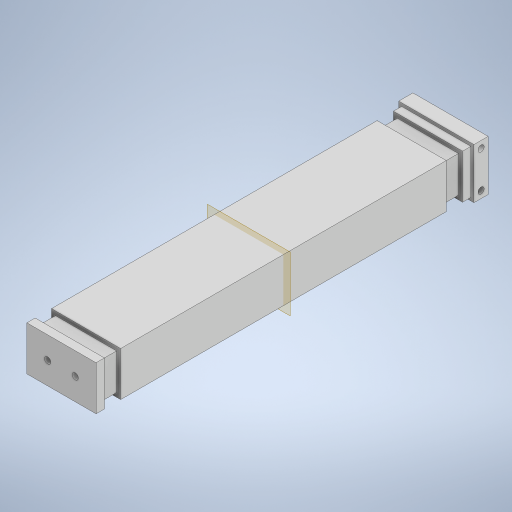
# Autodesk Inventor part: Mold
Saved by Autodesk Inventor 2024 (Build 280153000, 153)
## iProperties
Created: 2024-09-09
Part Number: Mold
Material: Generic
Document SubType Name: Modeling
Designer: Bruger
Density: 1 g/cm^3
Appearance: Default
Author: Bruger
Autodesk Inventor part; units mm, degrees
ref_plane "YZ Plane" through (0, 0, 0) normal (1, 0, 0) x (0, 1, 0)
ref_plane "XZ Plane" through (0, 0, 0) normal (0, 1, 0) x (-1, 0, 0)
ref_plane "XY Plane" through (0, 0, 0) normal (0, 0, 1) x (1, 0, 0)
sketch "Sketch8" plane through (0, 0, 0) normal (0, 0, 1) x (1, 0, 0)
  line L0 (-18.5, -12.375) -> (18.5, -12.375)
  line L1 (18.5, -12.375) -> (18.5, 12.375)
  line L2 (18.5, 12.375) -> (-18.5, 12.375)
  line L3 (-18.5, 12.375) -> (-18.5, -12.375)
  line L4 (-18.5, -12.375) -> (18.5, 12.375) construction
  line L5 (18.5, -12.375) -> (-18.5, 12.375) construction
  point P0 (0, 0)
  dimension "d43" = 37
  dimension "d44" = 24.75
  constraints: 12 end point, 2 midpoint, 2 parallel, 1 horizontal, 1 perpendicular
  measures "d43" distance of L2.end L1.end
  measures "d44" distance of L1.end L0.end
extrude "Extrusion6" add sketch "Sketch8" along normal blind 7
sketch "Sketch9" plane through (0, 0, 7) normal (0, 0, 1) x (1, 0, 0)
  line L0 (-17, -10.875) -> (17, -10.875)
  line L1 (17, -10.875) -> (17, 10.875)
  line L2 (17, 10.875) -> (-17, 10.875)
  line L3 (-17, 10.875) -> (-17, -10.875)
  line L4 (-17, -10.875) -> (17, 10.875) construction
  line L5 (17, -10.875) -> (-17, 10.875) construction
  line L6 (18.5, 12.375) -> (-18.5, 12.375) projected
  line L7 (18.5, -12.375) -> (18.5, 12.375) projected
  point P0 (0, 0)
  dimension "d49" = 1.5
  dimension "d50" = 1.5
  constraints: 12 end point, 2 midpoint, 2 parallel, 1 horizontal, 1 perpendicular
  measures "d49" distance between parallel lines of L6 L2
  measures "d50" distance between parallel lines of L7 L1
extrude "Extrusion7" add sketch "Sketch9" along normal blind 184.3
sketch "Sketch10" plane through (18.5, -12.375, 0) normal (1, 0, 0) x (0, 0, -1)
  circle A0 centre (-3.5, 21.325) radius 1.5
  line L0 (0, 0) -> (0, 24.75) projected
  line L1 (0, 24.75) -> (-7, 24.75) projected
  point P0 (0, 12.375)
  dimension "d53" = 3
  dimension "d56" = 3.425
  dimension "d57" = 3.5
  constraints: 1 centre point
  measures "d53" diameter of A0
  measures "d56" distance from line of L1 A0.centre
  measures "d57" distance from line of L0 A0.centre
hole "Hole1" at (18.5, 8.95, 3.5) direction (-1, 0, 0) diameter 3 depth 5 tip angle 118
mirror "Mirror1" about plane through (0, 0, 0) normal (0, 1, 0) of "Hole1"
mirror "Mirror2" about plane through (0, 0, 0) normal (1, 0, 0) of "Hole1", "Mirror1"
sketch "Sketch11" plane through (-18.5, -12.375, 0) normal (0, -1, 0) x (1, 0, 0)
  line L0 (18.5, 0) -> (18.5, 7)
  line L1 (37, 7) -> (0, 7) projected
  line L2 (18.5, 3.5) -> (0, 3.5)
  line L3 (0, 0) -> (0, 7) projected
  circle A0 centre (9.25, 3.5) radius 1.5
  dimension "d66" = 3
  constraints: 4 end point, 4 midpoint, 1 centre point
  measures "d66" diameter of A0
hole "Hole2" at (-9.25, -12.375, 3.5) direction (0, 1, 0) diameter 3 depth 5 tip angle 118
mirror "Mirror3" about plane through (0, 0, 0) normal (1, 0, 0) of "Hole2"
sketch "Sketch12" plane through (0, 0, 191.3) normal (0, 0, 1) x (1, 0, 0)
  circle A0 centre (6.8, 0) radius 1.5
  line L0 (17, -10.875) -> (17, 10.875) projected
  line L1 (17, 10.875) -> (-17, 10.875) projected
  point P0 (0, 0)
  dimension "d74" = 3
  dimension "d75" = 10.2
  dimension "d76" = 10.875
  constraints: 1 centre point
  measures "d74" diameter of A0
  measures "d75" distance from line of L0 A0.centre
  measures "d76" distance from line of L1 A0.centre
hole "Hole3" at (6.8, 0, 191.3) direction (0, 0, -1) diameter 3 depth 5 tip angle 118
mirror "Mirror4" about plane through (0, 0, 0) normal (1, 0, 0) of "Hole3"
sketch "Sketch13" plane through (-17, -10.875, 7) normal (-1, 0, 0) x (0, 0, 1)
  line L0 (0, 21.75) -> (4.1, 21.75)
  line L1 (0, 21.75) -> (184.3, 21.75) projected
  line L2 (4.1, 21.75) -> (4.1, 0)
  line L3 (0, 0) -> (184.3, 0) projected
  line L4 (4.1, 21.75) -> (12.1, 21.75)
  line L5 (0, 21.75) -> (184.3, 21.75) projected
  line L6 (12.1, 21.75) -> (12.1, 0)
  line L7 (12.1, 0) -> (4.1, 0)
  point P0 (-7, 10.875)
  dimension "d84" = 4.1
  dimension "d85" = 90
  dimension "d86" = 8
  dimension "d87" = 90
  constraints: 10 end point, 4 point on line
  measures "d84" distance of L0.start L0.end
  measures "d85" angle of L0 L2
  measures "d86" distance of L0.end L4.end
  measures "d87" angle of L4 L6
extrude "Extrusion8" cut sketch "Sketch13" against normal blind 2
mirror "Mirror5" about plane through (0, 0, 0) normal (1, 0, 0) of "Extrusion8"
sketch "Sketch14" plane through (-17, 10.875, 7) normal (0, 1, 0) x (1, 0, 0)
  line L0 (34, -4.1) -> (32, -4.1) projected
  line L1 (2, -4.1) -> (2, -12.1) projected
  line L2 (32, -4.1) -> (2, -4.1)
  line L3 (2, -4.1) -> (2, -12.1)
  line L4 (2, -12.1) -> (32, -12.1)
  line L5 (32, -12.1) -> (32, -4.1)
  point P0 (17, 7)
  constraints: 8 end point, 2 horizontal, 1 collinear, 1 perpendicular
extrude "Extrusion9" cut sketch "Sketch14" against normal blind 2
mirror "Mirror6" about plane through (0, 0, 0) normal (0, 1, 0) of "Extrusion9"
ref_plane "Work Plane4" through (0, 0, 99.15) normal (0, 0, 1) x (1, 0, 0)
mirror "Mirror7" about plane through (0, 0, 99.15) normal (0, 0, 1) of "Extrusion9", "Extrusion8", "Mirror5", "Mirror6"
body "Solid2"
